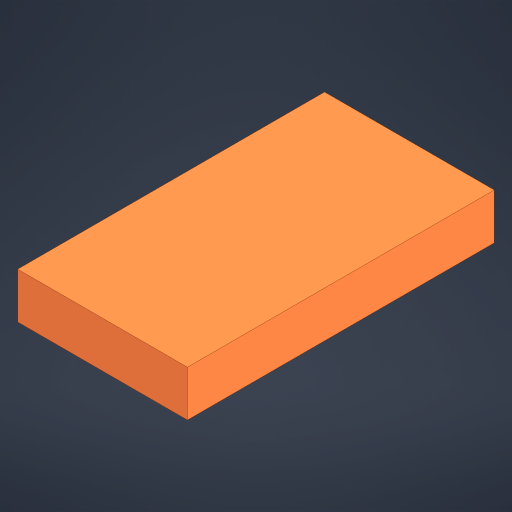
# Autodesk Inventor part: ESC
Saved by Autodesk Inventor 2024 (Build 280153000, 153)
## iProperties
Created: 2023-09-15
Part Number: ESC
Material: ESC
Document SubType Name: Modeling
Designer: Maciej
Mass: 21.9838 g
Surface Area: 34.66 cm^2
Volume: 8.554 cm^3
Density: 2.57 g/cm^3
Appearance: Generic
Author: Maciej
Autodesk Inventor part; units mm, degrees
ref_plane "YZ Plane" through (0, 0, 0) normal (1, 0, 0) x (0, 1, 0)
ref_plane "XZ Plane" through (0, 0, 0) normal (0, 1, 0) x (-1, 0, 0)
ref_plane "XY Plane" through (0, 0, 0) normal (0, 0, 1) x (1, 0, 0)
sketch "Sketch1" plane through (0, 0, 0) normal (0, 1, 0) x (-1, 0, 0)
  line L0 (13, 23.5) -> (-13, 23.5)
  line L1 (-13, 23.5) -> (-13, -23.5)
  line L2 (-13, -23.5) -> (13, -23.5)
  line L3 (13, -23.5) -> (13, 23.5)
  line L4 (13, 23.5) -> (-13, -23.5) construction
  line L5 (-13, 23.5) -> (13, -23.5) construction
  point P0 (0, 0)
  dimension "d0" = 26
  dimension "d1" = 47
  constraints: 12 end point, 2 midpoint, 2 parallel, 1 horizontal, 1 perpendicular
  measures "d0" distance of L2.end L1.end
  measures "d1" distance of L1.end L0.end
extrude "Extrusion1" add sketch "Sketch1" along normal blind 7
body "Solid1"
